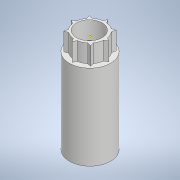
# Autodesk Inventor part: handle_base2
Saved by Autodesk Inventor 2021 (Build 250183000, 183)
## iProperties
Created: 2021-07-03
Part Number: handle_base2
Material: Generic
Document SubType Name: Modeling
Designer: teh18
Density: 1 g/cm^3
Appearance: Default
Author: teh18
Autodesk Inventor part; units mm, degrees
ref_plane "YZ Plane" through (0, 0, 0) normal (1, 0, 0) x (0, 1, 0)
ref_plane "XZ Plane" through (0, 0, 0) normal (0, 1, 0) x (-1, 0, 0)
ref_plane "XY Plane" through (0, 0, 0) normal (0, 0, 1) x (1, 0, 0)
sketch "Sketch4" plane through (0, 0, 0) normal (0, 1, 0) x (-1, 0, 0)
  point P0 (0, 0)
sketch "Sketch5" plane through (0, 0, 0) normal (0, 1, 0) x (-1, 0, 0)
  line L0 (-4.4351, -5.867) -> (-2.9352, -5.233) projected
  arc A0 (-2.9352, -5.233) -> (0.012, -6) centre (0, 0) ccw projected
  line L1 (0.012, -6) -> (1.0125, -7.2847) projected
  line L2 (1.0125, -7.2847) -> (1.6248, -5.7758) projected
  arc A1 (1.6248, -5.7758) -> (4.2511, -4.2342) centre (0, 0) ccw projected
  line L3 (4.2511, -4.2342) -> (5.867, -4.4351) projected
  line L4 (5.867, -4.4351) -> (5.233, -2.9352) projected
  arc A2 (5.233, -2.9352) -> (6, 0.012) centre (0, 0) ccw projected
  line L5 (6, 0.012) -> (7.2847, 1.0125) projected
  line L6 (7.2847, 1.0125) -> (5.7758, 1.6248) projected
  arc A3 (5.7758, 1.6248) -> (4.2342, 4.2511) centre (0, 0) ccw projected
  line L7 (4.2342, 4.2511) -> (4.4351, 5.867) projected
  line L8 (4.4351, 5.867) -> (2.9352, 5.233) projected
  arc A4 (2.9352, 5.233) -> (-0.012, 6) centre (0, 0) ccw projected
  line L9 (-0.012, 6) -> (-1.0125, 7.2847) projected
  line L10 (-1.0125, 7.2847) -> (-1.6248, 5.7758) projected
  arc A5 (-1.6248, 5.7758) -> (-4.2511, 4.2342) centre (0, 0) ccw projected
  line L11 (-4.2511, 4.2342) -> (-5.867, 4.4351) projected
  line L12 (-5.867, 4.4351) -> (-5.233, 2.9352) projected
  arc A6 (-5.233, 2.9352) -> (-6, -0.012) centre (0, 0) ccw projected
  line L13 (-6, -0.012) -> (-7.2847, -1.0125) projected
  line L14 (-7.2847, -1.0125) -> (-5.7758, -1.6248) projected
  arc A7 (-5.7758, -1.6248) -> (-4.2342, -4.2511) centre (0, 0) ccw projected
  line L15 (-4.2342, -4.2511) -> (-4.4351, -5.867) projected
  circle A8 centre (0.2493, 0.0186) radius 5 projected
  line L16 (5.1217, -2.9288) -> (5.7075, -4.3145)
  line L17 (5.7075, -4.3145) -> (4.2146, -4.1289)
  arc A9 (1.5507, -5.6926) -> (4.2146, -4.1289) centre (0, 0) ccw
  line L18 (1.5507, -5.6926) -> (0.985, -7.0866)
  line L19 (0.985, -7.0866) -> (0.0606, -5.8997)
  arc A10 (-2.9288, -5.1217) -> (0.0606, -5.8997) centre (0, 0) ccw
  line L20 (-2.9288, -5.1217) -> (-4.3145, -5.7075)
  line L21 (-4.3145, -5.7075) -> (-4.1289, -4.2146)
  arc A11 (-5.6926, -1.5507) -> (-4.1289, -4.2146) centre (0, 0) ccw
  line L22 (-5.6926, -1.5507) -> (-7.0866, -0.985)
  line L23 (-7.0866, -0.985) -> (-5.8997, -0.0606)
  arc A12 (-5.1217, 2.9288) -> (-5.8997, -0.0606) centre (0, 0) ccw
  line L24 (-5.1217, 2.9288) -> (-5.7075, 4.3145)
  line L25 (-5.7075, 4.3145) -> (-4.2146, 4.1289)
  arc A13 (-1.5507, 5.6926) -> (-4.2146, 4.1289) centre (0, 0) ccw
  line L26 (-1.5507, 5.6926) -> (-0.985, 7.0866)
  line L27 (-0.985, 7.0866) -> (-0.0606, 5.8997)
  arc A14 (2.9288, 5.1217) -> (-0.0606, 5.8997) centre (0, 0) ccw
  line L28 (2.9288, 5.1217) -> (4.3145, 5.7075)
  line L29 (4.3145, 5.7075) -> (4.1289, 4.2146)
  arc A15 (5.6926, 1.5507) -> (4.1289, 4.2146) centre (0, 0) ccw
  line L30 (5.6926, 1.5507) -> (7.0866, 0.985)
  line L31 (7.0866, 0.985) -> (5.8997, 0.0606)
  arc A16 (5.1217, -2.9288) -> (5.8997, 0.0606) centre (0, 0) ccw
  circle A17 centre (0, 0) radius 29.25 projected
  dimension "d22" = 0.1
  constraints: 32 end point, 16 point on circle, 8 centre point, 23 other
  measures "d22" distance between parallel lines of L4 L16
extrude "Extrusion4" add sketch "Sketch5" along normal blind 2 and the other way blind 5 contours L16 L17 A9 L18 L19 A10 L20 L21 A11 L22 L23 A12 L24 L25 A13 L26 L27 A14 L28 L29 A15 L30 L31 A16
sketch "Sketch6" plane through (0, -5, 0) normal (0, -1, 0) x (1, 0, 0)
  arc A0 (3.599, -4.8007) -> (5.4923, -2.4155) centre (0, 0) ccw projected
  arc A1 (0.8498, 5.9395) -> (-2.1756, 5.5917) centre (0, 0) ccw projected
  arc A2 (-4.8007, -3.599) -> (-2.4155, -5.4923) centre (0, 0) ccw projected
  arc A3 (-3.599, 4.8007) -> (-5.4923, 2.4155) centre (0, 0) ccw projected
  arc A4 (-0.8498, -5.9395) -> (2.1756, -5.5917) centre (0, 0) ccw projected
  arc A5 (5.9395, -0.8498) -> (5.5917, 2.1756) centre (0, 0) ccw projected
  arc A6 (-5.9395, 0.8498) -> (-5.5917, -2.1756) centre (0, 0) ccw projected
  arc A7 (4.8007, 3.599) -> (2.4155, 5.4923) centre (0, 0) ccw projected
  circle A8 centre (-0.2369, 0.08) radius 5 projected
  circle A9 centre (0, 0) radius 6
  circle A10 centre (0, 0) radius 8
  line L0 (2.1756, -5.5917) -> (3.5723, -6.4289) projected
  line L1 (3.5723, -6.4289) -> (3.599, -4.8007) projected
  line L2 (5.4923, -2.4155) -> (7.0719, -2.0199) projected
  line L3 (7.0719, -2.0199) -> (5.9395, -0.8498) projected
  line L4 (5.5917, 2.1756) -> (6.4289, 3.5723) projected
  line L5 (6.4289, 3.5723) -> (4.8007, 3.599) projected
  line L6 (2.4155, 5.4923) -> (2.0199, 7.0719) projected
  line L7 (2.0199, 7.0719) -> (0.8498, 5.9395) projected
  line L8 (-2.1756, 5.5917) -> (-3.5723, 6.4289) projected
  line L9 (-3.5723, 6.4289) -> (-3.599, 4.8007) projected
  line L10 (-5.4923, 2.4155) -> (-7.0719, 2.0199) projected
  line L11 (-7.0719, 2.0199) -> (-5.9395, 0.8498) projected
  line L12 (-5.5917, -2.1756) -> (-6.4289, -3.5723) projected
  line L13 (-6.4289, -3.5723) -> (-4.8007, -3.599) projected
  line L14 (-2.4155, -5.4923) -> (-2.0199, -7.0719) projected
  line L15 (-2.0199, -7.0719) -> (-0.8498, -5.9395) projected
  point P0 (0, 0)
  point P1 (2.1756, -5.5917)
  point P2 (-5.9204, 0.9738)
  point P3 (5.9395, -0.8498)
  point P4 (-4.875, -3.4978)
  point P5 (-2.3001, -5.5416)
  point P6 (-0.9738, -5.9204)
  point P7 (2.2921, -5.5449)
  point P8 (3.599, -4.8007)
  point P9 (5.4923, -2.4155)
  point P10 (0.8498, 5.9395)
  point P11 (-2.1756, 5.5917)
  point P12 (-4.8007, -3.599)
  point P13 (-2.4155, -5.4923)
  point P14 (-3.599, 4.8007)
  point P15 (-5.4923, 2.4155)
  point P16 (-0.8498, -5.9395)
  point P17 (-5.5917, -2.1756)
  point P18 (6, 0)
  point P19 (5.5917, 2.1756)
  point P20 (4.8007, 3.599)
  point P21 (2.4155, 5.4923)
  point P22 (-5.9395, 0.8498)
  dimension "d15" = 2
  constraints: 1 centre point, 1 coincident, 3 other
extrude "Extrusion5" add sketch "Sketch6" along normal blind 33 contours A9 A4 A2 A6 A3 A1 A7 A5 A0 | L1 L0 A9 | A9 L3 L2 | L15 L14 A9 | A9 L5 L4 | L13 L12 A9 | A9 L7 L6 | L11 L10 A9 | A9 L9 L8 | A10
sketch "Sketch8" plane through (0, -38, 0) normal (0, -1, 0) x (1, 0, 0)
  circle A0 centre (0, 0) radius 8 projected
  circle A1 centre (0, 0) radius 6.1
  point P0 (0, 0)
  dimension "d19" = 12.2
  constraints: 1 centre point, 1 coincident
  measures "d19" diameter of A1
extrude "Extrusion7" cut sketch "Sketch8" against normal blind 10 contours A1
body "Solid2"
